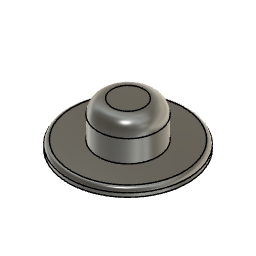
Hat (Autodesk Fusion 360 design; units mm, degrees)
Autodesk Fusion 360 part; units mm, degrees
sketch "Sketch2" plane through (0, 0, 0) normal (0, 0, 1) x (1, 0, 0)
  circle A0 centre (0, 0) radius 38.1
  dimension "d15" = 76.2
  constraint coincident A0.centre origin
  measures "d15" diameter of A0
extrude "Extrude1" add sketch "Sketch2" along normal blind 5
sketch "Sketch3" plane through (0, 0, 5) normal (0, 0, 1) x (-1, 0, 0)
  circle A0 centre (0, 0) radius 38.1
  circle A1 centre (0, 0) radius 19.05
  dimension "d14" = 38.1
  constraint concentric A0 A1
  measures "d14" diameter of A1
extrude "Extrude2" add sketch "Sketch3" along normal blind 22.86 contours A1
sketch "Sketch4" plane through (0, 0, 0) normal (0, 0, -1) x (1, 0, 0)
  circle A0 centre (0, 0) radius 38.1
  circle A1 centre (0.0969, -12.6996) radius 2.2098
  circle A2 centre (10.9498, 6.4337) radius 2.2098
  circle A3 centre (-11.0466, 6.2659) radius 2.2098
  arc A4 (2.2968, -12.4906) -> (11.8992, 4.4383) centre (0, 0) ccw
  arc A5 (9.6688, 8.2343) -> (-9.7933, 8.0859) centre (0, 0) ccw
  arc A6 (-11.9656, 4.2562) -> (-2.106, -12.5242) centre (0, 0) ccw
  dimension "d7" = 4.4196
  dimension "d9" = 360
  constraint coincident A0.centre A4.centre
  constraint coincident A1.centre A4
  constraint coincident A1 A6.end
  constraint coincident A1 A4.start
  constraint coincident A2 A4.end
  constraint coincident A2 A5.start
  constraint concentric A4 A5
  constraint coincident A3 A5.end
  constraint coincident A3 A6.start
  constraint concentric A5 A6
  measures "d7" diameter of A1
extrude "Extrude3" add sketch "Sketch4" along normal blind 5 contours A1 | A2 | A3
fillet "Fillet2" radius 8.89 1 edges at (17.7608, 6.8888, 27.86)
fillet "Fillet3" radius 2.54 1 edges at (-35.5217, -13.7775, 5)
